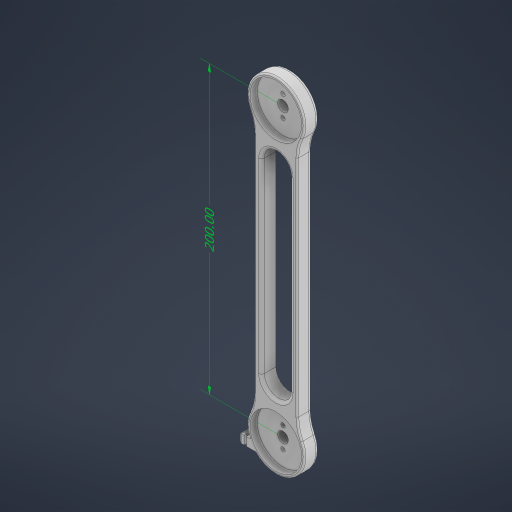
# Autodesk Inventor part: Arm 01-large
Saved by Autodesk Inventor 2023 (Build 270158000, 158)
## iProperties
Created: 2023-09-23
Part Number: Arm 01-large
Material: Generic
Document SubType Name: Modeling
Designer: hrush
Density: 1 g/cm^3
Appearance: Default
Mass: 34.2117 g
Surface Area: 182.829 cm^2
Volume: 34.2117 cm^3
Author: hrush
Autodesk Inventor part; units mm, degrees
ref_plane "YZ Plane" through (0, 0, 0) normal (1, 0, 0) x (0, 1, 0)
ref_plane "XZ Plane" through (0, 0, 0) normal (0, 1, 0) x (-1, 0, 0)
ref_plane "XY Plane" through (0, 0, 0) normal (0, 0, 1) x (1, 0, 0)
sketch "Sketch1" plane through (0, 0, 0) normal (0, 0, 1) x (1, 0, 0)
  arc A0 (-18, 8.7178) -> (18, 8.7178) centre (0, 0) ccw
  line L0 (15, 21.7945) -> (15, 178.2055)
  line L1 (-15, 178.2055) -> (-15, 21.7945)
  arc A1 (18, 191.2822) -> (-18, 191.2822) centre (0, 200) ccw
  arc A2 (-18, 8.7178) -> (-15, 21.7945) centre (-45, 21.7945) ccw
  arc A3 (15, 21.7945) -> (18, 8.7178) centre (45, 21.7945) ccw
  arc A4 (-15, 178.2055) -> (-18, 191.2822) centre (-45, 178.2055) ccw
  arc A5 (18, 191.2822) -> (15, 178.2055) centre (45, 178.2055) ccw
  line L2 (-15, -13.2288) -> (-25, -13.2288)
  line L3 (-25, -13.2288) -> (-25, -7.2288)
  line L4 (-25, -7.2288) -> (-18.6479, -7.2288)
  point P0 (-15, 13.2288)
  point P1 (15, 13.2288)
  point P2 (-15, 186.7712)
  point P3 (15, 186.7712)
  dimension "d0" = 40
  dimension "d3" = 40
  dimension "d4" = 30
  constraints: 18 point on circle, 10 end point, 8 tangent, 6 centre point, 4 point on line, 3 equal radius, 2 parallel, 1 coincident, 1 horizontal, 1 perpendicular
  measures "d0" diameter of A0
  measures "d3" diameter of A1
  measures "d4" radius of A2
extrude "Extrusion1" add sketch "Sketch1" along normal blind 10
sketch "Sketch2" plane through (0, 0, 10) normal (0, 0, 1) x (1, 0, 0)
  circle A0 centre (0, 0) radius 3.75
  circle A1 centre (0, 7.25) radius 1.5
  circle A2 centre (0, -7.25) radius 1.5
  circle A3 centre (0, 200) radius 3.75
  circle A4 centre (0, 207.25) radius 1.5
  circle A5 centre (0, 192.75) radius 1.5
  dimension "d7" = 7.5
  dimension "d8" = 3
  dimension "d9" = 3
  dimension "d10" = 7.25
  dimension "d11" = 7.25
  dimension "d12" = 7.5
  dimension "d13" = 3
  dimension "d14" = 3
  dimension "d15" = 7.25
  dimension "d16" = 7.25
  constraints: 6 centre point, 1 coincident
  measures "d7" diameter of A0
  measures "d8" diameter of A1
  measures "d9" diameter of A2
  measures "d10" distance of point (0, 0) A1.centre
  measures "d11" distance of point (0, 0) A2.centre
  measures "d12" diameter of A3
  measures "d13" diameter of A4
  measures "d14" diameter of A5
  measures "d15" distance of A3.centre A4.centre
  measures "d16" distance of A3.centre A5.centre
extrude "Extrusion2" cut sketch "Sketch2" against normal blind 10
sketch "Sketch3" plane through (0, 0, 10) normal (0, 0, 1) x (1, 0, 0)
  circle A0 centre (0, 0) radius 18
  circle A1 centre (0, 200) radius 18
  dimension "d19" = 36
  dimension "d20" = 36
  constraints: 2 centre point, 1 coincident
  measures "d19" diameter of A0
  measures "d20" diameter of A1
extrude "Extrusion3" cut sketch "Sketch3" against normal blind 5
sketch "Sketch4" plane through (0, 0, 10) normal (0, 0, 1) x (1, 0, 0)
  line L0 (-10, 175) -> (10, 175)
  line L1 (10, 175) -> (10, 25)
  line L2 (10, 25) -> (-10, 25)
  line L3 (-10, 25) -> (-10, 175)
  line L4 (-15, 178.2055) -> (-15, 21.7945) projected
  point P0 (0, 0)
  dimension "d23" = 20
  dimension "d24" = 150
  dimension "d32" = 5
  constraints: 8 end point, 2 parallel, 1 horizontal, 1 perpendicular
  measures "d23" distance of L1.end L2.end
  measures "d24" distance of L0.end L1.end
  measures "d32" distance between parallel lines of L4 L3
extrude "Extrusion4" cut sketch "Sketch4" against normal blind 10
fillet "Fillet1" radius 10 4 edges at (-10, 175, 5) (10, 175, 5) (-10, 25, 5) (10, 25, 5)
sketch "Sketch6" plane through (-25, -7.2288, 0) normal (0, 1, 0) x (1, 0, 0)
  line L0 (1.4955, -8.3045) -> (4.499, -8.3045)
  line L1 (4.499, -8.3045) -> (4.499, -2.8798)
  line L2 (4.499, -2.8798) -> (1.4955, -2.8798)
  line L3 (1.4955, -2.8798) -> (1.4955, -8.3045)
  line L4 (2.9973, -8.3045) -> (4.499, -8.3045)
  line L5 (4.499, -8.3045) -> (4.499, -10.2532)
  line L6 (4.499, -10.2532) -> (2.9973, -10.2532)
  line L7 (2.9973, -10.2532) -> (2.9973, -8.3045)
  point P0 (25, 0)
  constraints: 16 end point, 4 parallel, 2 horizontal, 2 perpendicular, 1 midpoint
extrude "Extrusion5" cut sketch "Sketch6" against normal blind 10
fillet "Fillet2" radius 1 9 edges at (-15.7596, 15.0863, 10) (-19.9835, 0.8119, 10) (-15.7596, 184.9137, 10) (0, 220, 10) (15.7596, 184.9137, 10) (15, 100, 10) (15.7596, 15.0863, 10) (11.0753, -16.6534, 10) (-15, 100, 10)
fillet "Fillet3" radius 2 4 edges at (-7.0711, 27.9289, 10) (-10, 100, 10) (-7.0711, 172.0711, 10) (10, 100, 10)
fillet "Fillet4" radius 2 9 edges at (15.7596, 184.9137, 0) (0, 220, 0) (-15.7596, 184.9137, 0) (-15, 100, 0) (-15.7596, 15.0863, 0) (-19.9835, 0.8119, 0) (15.7596, 15.0863, 0) (11.0753, -16.6534, 0) (15, 100, 0)
fillet "Fillet5" radius 1 3 edges at (-25, -7.2288, 5) (-25, -13.2288, 5) (-25, -10.2288, 10)
body "Solid1"
